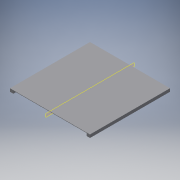
# Autodesk Inventor part: Alum Bed plate
Saved by Autodesk Inventor 2016 (Build 200138000, 138)
## iProperties
Created: 2016-05-26
Part Number: Alum Bed plate
Material: Generic
Document SubType Name: Modeling
Designer: Scott
Density: 1 g/cm^3
Appearance: Default
Author: Scott
Autodesk Inventor part; units mm, degrees
ref_plane "YZ Plane" through (0, 0, 0) normal (1, 0, 0) x (0, 1, 0)
ref_plane "XZ Plane" through (0, 0, 0) normal (0, 1, 0) x (-1, 0, 0)
ref_plane "XY Plane" through (0, 0, 0) normal (0, 0, 1) x (1, 0, 0)
sketch "Sketch2" plane through (0, 0, 0) normal (0, 1, 0) x (-1, 0, 0)
  line L0 (-304.8, -304.8) -> (304.8, -304.8)
  line L1 (304.8, -304.8) -> (304.8, 304.8)
  line L2 (304.8, 304.8) -> (-304.8, 304.8)
  line L3 (-304.8, 304.8) -> (-304.8, -304.8)
  line L4 (-304.8, -304.8) -> (304.8, 304.8) construction
  line L5 (304.8, -304.8) -> (-304.8, 304.8) construction
  point P0 (0, 0)
  dimension "d4" = 609.6
  dimension "d5" = 609.6
  constraints: 12 end point, 2 midpoint, 2 parallel, 1 horizontal, 1 perpendicular
  measures "d4" distance of L2.end L1.end
  measures "d5" distance of L1.end L0.end
extrude "Extrusion2" add sketch "Sketch2" along normal blind 3.175
sketch "Sketch3" plane through (0, 3.175, 0) normal (0, 1, 0) x (1, 0, 0)
  line L0 (304.8, 304.8) -> (-304.8, 304.8) projected
  line L1 (-304.8, -304.8) -> (304.8, -304.8) projected
  line L2 (-304.8, 304.8) -> (-279.4, 304.8)
  line L3 (-279.4, 304.8) -> (-279.4, -304.8)
  line L4 (-279.4, -304.8) -> (-304.8, -304.8)
  line L5 (-304.8, -304.8) -> (-304.8, 304.8)
  line L6 (304.8, 304.8) -> (279.4, 304.8)
  line L7 (279.4, 304.8) -> (279.4, -304.8)
  line L8 (279.4, -304.8) -> (304.8, -304.8)
  line L9 (304.8, -304.8) -> (304.8, 304.8)
  line L10 (304.8, 304.8) -> (-304.8, 304.8) projected
  line L11 (304.8, -304.8) -> (304.8, 304.8) projected
  line L12 (-304.8, -304.8) -> (304.8, -304.8) projected
  line L13 (-304.8, 304.8) -> (-304.8, -304.8) projected
  line L14 (-304.8, -304.8) -> (-279.4, -304.8)
  line L15 (-279.4, -304.8) -> (-279.4, 318.078)
  line L16 (-279.4, 318.078) -> (-304.8, 318.078)
  line L17 (-304.8, 318.078) -> (-304.8, -304.8)
  line L18 (304.8, -304.8) -> (304.8, 304.8) projected
  line L19 (304.8, -304.8) -> (279.4, -304.8)
  line L20 (279.4, -304.8) -> (279.4, 304.8)
  line L21 (279.4, 304.8) -> (304.8, 304.8)
  line L22 (304.8, 304.8) -> (304.8, -304.8)
  line L23 (-304.8, 304.8) -> (-304.8, -304.8) projected
  line L24 (-304.8, -304.8) -> (-279.4, -304.8)
  line L25 (-279.4, -304.8) -> (-279.4, 304.8)
  line L26 (-279.4, 304.8) -> (-304.8, 304.8)
  line L27 (-304.8, 304.8) -> (-304.8, -304.8)
  point P0 (0, 0)
  dimension "d8" = 25.4
  dimension "d9" = 25.4
  constraints: 40 end point, 10 parallel, 5 horizontal, 5 perpendicular, 3 point on line
  measures "d8" distance of L3.end L4.end
  measures "d9" distance of L8.end L7.end
extrude "Extrusion3" add sketch "Sketch3" against normal blind 23.175 contours L9 L1 L7 L0 | L3 L1 L5 L0
ref_plane "Work Plane1" through (0, 3.175, 304.8) normal (1, 0, 0) x (0, 0, -1)
body "Solid2"
